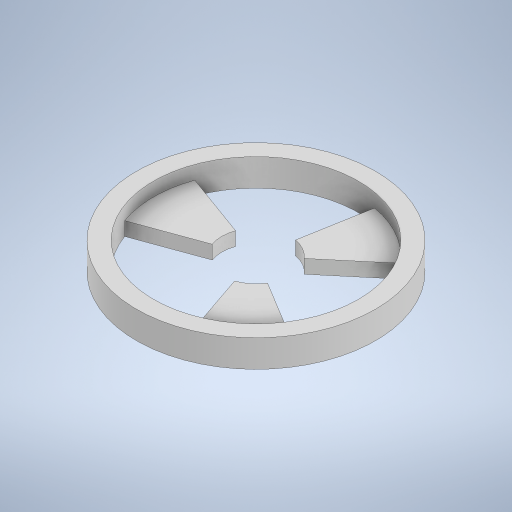
# Autodesk Inventor part: fan_num5_1
Saved by Autodesk Inventor 2024 (Build 280153000, 153)
## iProperties
Created: 2024-08-06
Part Number: fan_num5_1
Material: 일반
Document SubType Name: Modeling
Designer: chlqj
Density: 1 g/cm^3
Appearance: 기본값
Author: chlqj
Autodesk Inventor part; units mm, degrees
ref_plane "YZ Plane" through (0, 0, 0) normal (1, 0, 0) x (0, 1, 0)
ref_plane "XZ Plane" through (0, 0, 0) normal (0, 1, 0) x (-1, 0, 0)
ref_plane "XY Plane" through (0, 0, 0) normal (0, 0, 1) x (1, 0, 0)
sketch "스케치1" plane through (0, 0, 0) normal (0, 1, 0) x (-1, 0, 0)
  circle A0 centre (0, 0) radius 15
  circle A1 centre (0, 0) radius 17.5
  dimension "d0" = 30
  dimension "d1" = 35
  constraints: 2 centre point, 2 coincident
  measures "d0" diameter of A0
  measures "d1" diameter of A1
extrude "돌출1" add sketch "스케치1" along normal blind 2
sketch "스케치2" plane through (0, 2, 0) normal (0, 1, 0) x (1, 0, 0)
  line L0 (0, 0) -> (-15, 0)
  circle A0 centre (0, 0) radius 15 projected
  line L1 (0, 0) -> (-14.0954, -5.1303)
  line L2 (0, 0) -> (15, 0) construction
  line L3 (0, 0) -> (-14.0954, 5.1303)
  line L4 (0, 0) -> (11.4907, 9.6418)
  line L5 (0, 0) -> (2.6047, 14.7721)
  line L6 (0, 0) -> (12.8233, -7.7822)
  line L7 (0, 0) -> (4.8209, -14.2042)
  arc A1 (-14.0954, 5.1303) -> (-14.0954, -5.1303) centre (0, 0) ccw
  arc A2 (4.8209, -14.2042) -> (12.8233, -7.7822) centre (0, 0) ccw
  arc A3 (11.4907, 9.6418) -> (2.6047, 14.7721) centre (0, 0) ccw
  circle A4 centre (0, 0) radius 5
  point P0 (-7.5, 0)
  point P1 (0.8682, 4.924)
  point P2 (3.8302, 3.2139)
  point P3 (4.2744, -2.5941)
  point P4 (1.607, -4.7347)
  point P5 (-4.6985, 1.7101)
  point P6 (-4.6985, -1.7101)
  dimension "d15" = 10
  constraints: 16 end point, 6 point on circle, 4 centre point, 2 horizontal, 1 coincident, 1 equal length, 1 midpoint, 11 other
  measures "d15" diameter of A4
extrude "돌출2" add sketch "스케치2" against normal blind 2 contours A4 L1 A0 L0 | L0 A0 L3 A4 | A4 L5 A0 L4 | L6 A0 L7 A4
sketch "스케치3" plane through (0, 2, 0) normal (0, 1, 0) x (1, 0, 0)
  circle A0 centre (0, 0) radius 15
  circle A1 centre (0, 0) radius 17.5
  dimension "d18" = 30
  constraints: 2 centre point, 2 coincident
  measures "d18" diameter of A0
extrude "돌출3" add sketch "스케치3" along normal blind 2
